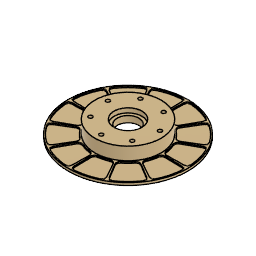
Brodie Stator Top (Autodesk Fusion 360 design; units mm, degrees)
Autodesk Fusion 360 part; units mm, degrees
sketch "Sketch1" plane through (0, 0, 0) normal (0, 0, 1) x (1, 0, 0)
  circle A0 centre (0, 0) radius 26
  circle A1 centre (0, 0) radius 47
  dimension "d1" = 52
  dimension "d2" = 94
  constraint coincident A0.centre A1.centre
  measures "d1" diameter of A0
  measures "d2" diameter of A1
extrude "Extrude1" add sketch "Sketch1" along normal blind 2 contours A0 | A1
sketch "Sketch2" plane through (0, 0, 2) normal (0, 0, 1) x (-1, 0, 0)
  circle A0 centre (0, 0) radius 47
  circle A1 centre (0, 0) radius 26
  constraint coincident A0.centre A1.centre
extrude "Extrude2" add sketch "Sketch2" along normal blind 10 contours A1
sketch "Sketch3" plane through (0, 0, 0) normal (0, 0, -1) x (1, 0, 0)
  circle A0 centre (0, 0) radius 47
  circle A1 centre (0, 0) radius 24
  constraint concentric A0 A1
extrude "Extrude3" cut sketch "Sketch3" against normal blind 3.5 contours A1
sketch "Sketch4" plane through (0, 0, 3.5) normal (0, 0, -1) x (1, 0, 0)
  circle A0 centre (0, 0) radius 24
  circle A1 centre (0, 0) radius 8.5
  dimension "d9" = 17
  constraint concentric A0 A1
  measures "d9" diameter of A1
extrude "Extrude4" cut sketch "Sketch4" against normal blind 31 contours A1
sketch "Sketch5" plane through (0, 0, 12) normal (0, 0, 1) x (-1, 0, 0)
  circle A0 centre (0, 0) radius 8.5
  circle A1 centre (0, 0) radius 26
  circle A2 centre (0, 0) radius 11
  constraint coincident A0.centre A1.centre
extrude "Extrude5" cut sketch "Sketch5" against normal blind 3.5 contours A2
sketch "Sketch6" plane through (0, 0, 3.5) normal (0, 0, -1) x (1, 0, 0)
  circle A0 centre (0, 0) radius 8.5
  circle A1 centre (0, 0) radius 24
  circle A2 centre (0, 0) radius 18
  constraint coincident A0.centre A1.centre
extrude "Extrude6" add sketch "Sketch6" along normal blind 1.5 contours A1
sketch "Sketch7" plane through (0, 0, 2) normal (0, 0, -1) x (1, 0, 0)
  circle A0 centre (0, 0) radius 18
  circle A1 centre (0, 0) radius 24
  circle A2 centre (0, 21) radius 1.5
  circle A3 centre (-16.4185, 13.0933) radius 1.5
  circle A4 centre (-20.4735, -4.6729) radius 1.5
  circle A5 centre (-9.1116, -18.9203) radius 1.5
  circle A6 centre (9.1116, -18.9203) radius 1.5
  circle A7 centre (20.4735, -4.6729) radius 1.5
  circle A8 centre (16.4185, 13.0933) radius 1.5
  dimension "d16" = 3
  dimension "d18" = 360
  measures "d16" diameter of A2
extrude "Extrude7" cut sketch "Sketch7" against normal blind 10 contours A2 | A3 | A4 | A5 | A6 | A7 | A8
sketch "Sketch8" plane through (0, 0, 2) normal (0, 0, 1) x (-1, 0, 0)
  circle A0 centre (0, 0) radius 26
  circle A1 centre (0, 0) radius 47
  line L0 (-0.5209, -29.8451) -> (-0.7486, -42.8887)
  line L1 (-14.4714, -26.1071) -> (-20.796, -37.517)
  arc A2 (-19.44, -41.6904) -> (-4.0097, -45.8249) centre (0, 0) ccw
  arc A3 (-10.6628, -24.8053) -> (-3.1684, -26.8134) centre (0, 0) ccw
  arc A4 (-4.0097, -45.8249) -> (-0.7486, -42.8887) centre (-3.7482, -42.8363) ccw
  arc A5 (-20.796, -37.517) -> (-19.44, -41.6904) centre (-18.1722, -38.9714) ccw
  arc A6 (-0.5209, -29.8451) -> (-3.1684, -26.8134) centre (-3.5205, -29.7927) ccw
  arc A7 (-10.6628, -24.8053) -> (-14.4714, -26.1071) centre (-11.8475, -27.5615) ccw
  arc A8 (-21.1397, -39.4118) -> (-20.8317, -40.3595) centre (-21.0253, -39.8985) ccw
  arc A9 (-2.139, -45.3682) -> (-1.3984, -44.7014) centre (-1.7408, -45.0658) ccw
  arc A10 (4.0097, -45.8249) -> (19.44, -41.6904) centre (0, 0) ccw
  arc A11 (0.7486, -42.8887) -> (4.0097, -45.8249) centre (3.7482, -42.8363) ccw
  arc A12 (1.3984, -44.7014) -> (2.139, -45.3682) centre (1.7408, -45.0658) ccw
  line L2 (0.5209, -29.8451) -> (0.7486, -42.8887)
  arc A13 (3.1684, -26.8134) -> (0.5209, -29.8451) centre (3.5205, -29.7927) ccw
  arc A14 (3.1684, -26.8134) -> (10.6628, -24.8053) centre (0, 0) ccw
  arc A15 (14.4714, -26.1071) -> (10.6628, -24.8053) centre (11.8475, -27.5615) ccw
  line L3 (14.4714, -26.1071) -> (20.796, -37.517)
  arc A16 (19.44, -41.6904) -> (20.796, -37.517) centre (18.1722, -38.9714) ccw
  arc A17 (20.8317, -40.3595) -> (21.1397, -39.4118) centre (21.0253, -39.8985) ccw
  arc A18 (26.3849, -37.6807) -> (37.6807, -26.3849) centre (0, 0) ccw
  arc A19 (22.0927, -36.7684) -> (26.3849, -37.6807) centre (24.6642, -35.2233) ccw
  arc A20 (23.5617, -38.0134) -> (24.5365, -38.2205) centre (24.0405, -38.1577) ccw
  line L4 (15.3737, -25.5861) -> (22.0927, -36.7684)
  arc A21 (16.1507, -21.6369) -> (15.3737, -25.5861) centre (17.9452, -24.041) ccw
  arc A22 (16.1507, -21.6369) -> (21.6369, -16.1507) centre (0, 0) ccw
  arc A23 (25.5861, -15.3737) -> (21.6369, -16.1507) centre (24.041, -17.9452) ccw
  line L5 (25.5861, -15.3737) -> (36.7684, -22.0927)
  arc A24 (37.6807, -26.3849) -> (36.7684, -22.0927) centre (35.2233, -24.6642) ccw
  arc A25 (38.2205, -24.5365) -> (38.0134, -23.5617) centre (38.1577, -24.0405) ccw
  arc A26 (41.6904, -19.44) -> (45.8249, -4.0097) centre (0, 0) ccw
  arc A27 (37.517, -20.796) -> (41.6904, -19.44) centre (38.9714, -18.1722) ccw
  arc A28 (39.4118, -21.1397) -> (40.3595, -20.8317) centre (39.8985, -21.0253) ccw
  line L6 (26.1071, -14.4714) -> (37.517, -20.796)
  arc A29 (24.8053, -10.6628) -> (26.1071, -14.4714) centre (27.5615, -11.8475) ccw
  arc A30 (24.8053, -10.6628) -> (26.8134, -3.1684) centre (0, 0) ccw
  arc A31 (29.8451, -0.5209) -> (26.8134, -3.1684) centre (29.7927, -3.5205) ccw
  line L7 (29.8451, -0.5209) -> (42.8887, -0.7486)
  arc A32 (45.8249, -4.0097) -> (42.8887, -0.7486) centre (42.8363, -3.7482) ccw
  arc A33 (45.3682, -2.139) -> (44.7014, -1.3984) centre (45.0658, -1.7408) ccw
  arc A34 (45.8249, 4.0097) -> (41.6904, 19.44) centre (0, 0) ccw
  arc A35 (42.8887, 0.7486) -> (45.8249, 4.0097) centre (42.8363, 3.7482) ccw
  arc A36 (44.7014, 1.3984) -> (45.3682, 2.139) centre (45.0658, 1.7408) ccw
  line L8 (29.8451, 0.5209) -> (42.8887, 0.7486)
  arc A37 (26.8134, 3.1684) -> (29.8451, 0.5209) centre (29.7927, 3.5205) ccw
  arc A38 (26.8134, 3.1684) -> (24.8053, 10.6628) centre (0, 0) ccw
  arc A39 (26.1071, 14.4714) -> (24.8053, 10.6628) centre (27.5615, 11.8475) ccw
  line L9 (26.1071, 14.4714) -> (37.517, 20.796)
  arc A40 (41.6904, 19.44) -> (37.517, 20.796) centre (38.9714, 18.1722) ccw
  arc A41 (40.3595, 20.8317) -> (39.4118, 21.1397) centre (39.8985, 21.0253) ccw
  arc A42 (37.6807, 26.3849) -> (26.3849, 37.6807) centre (0, 0) ccw
  arc A43 (36.7684, 22.0927) -> (37.6807, 26.3849) centre (35.2233, 24.6642) ccw
  arc A44 (38.0134, 23.5617) -> (38.2205, 24.5365) centre (38.1577, 24.0405) ccw
  line L10 (25.5861, 15.3737) -> (36.7684, 22.0927)
  arc A45 (21.6369, 16.1507) -> (25.5861, 15.3737) centre (24.041, 17.9452) ccw
  arc A46 (21.6369, 16.1507) -> (16.1507, 21.6369) centre (0, 0) ccw
  arc A47 (15.3737, 25.5861) -> (16.1507, 21.6369) centre (17.9452, 24.041) ccw
  line L11 (15.3737, 25.5861) -> (22.0927, 36.7684)
  arc A48 (26.3849, 37.6807) -> (22.0927, 36.7684) centre (24.6642, 35.2233) ccw
  arc A49 (24.5365, 38.2205) -> (23.5617, 38.0134) centre (24.0405, 38.1577) ccw
  arc A50 (19.44, 41.6904) -> (4.0097, 45.8249) centre (0, 0) ccw
  arc A51 (20.796, 37.517) -> (19.44, 41.6904) centre (18.1722, 38.9714) ccw
  arc A52 (21.1397, 39.4118) -> (20.8317, 40.3595) centre (21.0253, 39.8985) ccw
  line L12 (14.4714, 26.1071) -> (20.796, 37.517)
  arc A53 (10.6628, 24.8053) -> (14.4714, 26.1071) centre (11.8475, 27.5615) ccw
  arc A54 (10.6628, 24.8053) -> (3.1684, 26.8134) centre (0, 0) ccw
  arc A55 (0.5209, 29.8451) -> (3.1684, 26.8134) centre (3.5205, 29.7927) ccw
  line L13 (0.5209, 29.8451) -> (0.7486, 42.8887)
  arc A56 (4.0097, 45.8249) -> (0.7486, 42.8887) centre (3.7482, 42.8363) ccw
  arc A57 (2.139, 45.3682) -> (1.3984, 44.7014) centre (1.7408, 45.0658) ccw
  arc A58 (-4.0097, 45.8249) -> (-19.44, 41.6904) centre (0, 0) ccw
  arc A59 (-0.7486, 42.8887) -> (-4.0097, 45.8249) centre (-3.7482, 42.8363) ccw
  arc A60 (-1.3984, 44.7014) -> (-2.139, 45.3682) centre (-1.7408, 45.0658) ccw
  line L14 (-0.5209, 29.8451) -> (-0.7486, 42.8887)
  arc A61 (-3.1684, 26.8134) -> (-0.5209, 29.8451) centre (-3.5205, 29.7927) ccw
  arc A62 (-3.1684, 26.8134) -> (-10.6628, 24.8053) centre (0, 0) ccw
  arc A63 (-14.4714, 26.1071) -> (-10.6628, 24.8053) centre (-11.8475, 27.5615) ccw
  line L15 (-14.4714, 26.1071) -> (-20.796, 37.517)
  arc A64 (-19.44, 41.6904) -> (-20.796, 37.517) centre (-18.1722, 38.9714) ccw
  arc A65 (-20.8317, 40.3595) -> (-21.1397, 39.4118) centre (-21.0253, 39.8985) ccw
  arc A66 (-26.3849, 37.6807) -> (-37.6807, 26.3849) centre (0, 0) ccw
  arc A67 (-22.0927, 36.7684) -> (-26.3849, 37.6807) centre (-24.6642, 35.2233) ccw
  arc A68 (-23.5617, 38.0134) -> (-24.5365, 38.2205) centre (-24.0405, 38.1577) ccw
  line L16 (-15.3737, 25.5861) -> (-22.0927, 36.7684)
  arc A69 (-16.1507, 21.6369) -> (-15.3737, 25.5861) centre (-17.9452, 24.041) ccw
  arc A70 (-16.1507, 21.6369) -> (-21.6369, 16.1507) centre (0, 0) ccw
  arc A71 (-25.5861, 15.3737) -> (-21.6369, 16.1507) centre (-24.041, 17.9452) ccw
  line L17 (-25.5861, 15.3737) -> (-36.7684, 22.0927)
  arc A72 (-37.6807, 26.3849) -> (-36.7684, 22.0927) centre (-35.2233, 24.6642) ccw
  arc A73 (-38.2205, 24.5365) -> (-38.0134, 23.5617) centre (-38.1577, 24.0405) ccw
  arc A74 (-41.6904, 19.44) -> (-45.8249, 4.0097) centre (0, 0) ccw
  arc A75 (-37.517, 20.796) -> (-41.6904, 19.44) centre (-38.9714, 18.1722) ccw
  arc A76 (-39.4118, 21.1397) -> (-40.3595, 20.8317) centre (-39.8985, 21.0253) ccw
  line L18 (-26.1071, 14.4714) -> (-37.517, 20.796)
  arc A77 (-24.8053, 10.6628) -> (-26.1071, 14.4714) centre (-27.5615, 11.8475) ccw
  arc A78 (-24.8053, 10.6628) -> (-26.8134, 3.1684) centre (0, 0) ccw
  arc A79 (-29.8451, 0.5209) -> (-26.8134, 3.1684) centre (-29.7927, 3.5205) ccw
  line L19 (-29.8451, 0.5209) -> (-42.8887, 0.7486)
  arc A80 (-45.8249, 4.0097) -> (-42.8887, 0.7486) centre (-42.8363, 3.7482) ccw
  arc A81 (-45.3682, 2.139) -> (-44.7014, 1.3984) centre (-45.0658, 1.7408) ccw
  arc A82 (-45.8249, -4.0097) -> (-41.6904, -19.44) centre (0, 0) ccw
  arc A83 (-42.8887, -0.7486) -> (-45.8249, -4.0097) centre (-42.8363, -3.7482) ccw
  arc A84 (-44.7014, -1.3984) -> (-45.3682, -2.139) centre (-45.0658, -1.7408) ccw
  line L20 (-29.8451, -0.5209) -> (-42.8887, -0.7486)
  arc A85 (-26.8134, -3.1684) -> (-29.8451, -0.5209) centre (-29.7927, -3.5205) ccw
  arc A86 (-26.8134, -3.1684) -> (-24.8053, -10.6628) centre (0, 0) ccw
  arc A87 (-26.1071, -14.4714) -> (-24.8053, -10.6628) centre (-27.5615, -11.8475) ccw
  line L21 (-26.1071, -14.4714) -> (-37.517, -20.796)
  arc A88 (-41.6904, -19.44) -> (-37.517, -20.796) centre (-38.9714, -18.1722) ccw
  arc A89 (-40.3595, -20.8317) -> (-39.4118, -21.1397) centre (-39.8985, -21.0253) ccw
  arc A90 (-37.6807, -26.3849) -> (-26.3849, -37.6807) centre (0, 0) ccw
  arc A91 (-36.7684, -22.0927) -> (-37.6807, -26.3849) centre (-35.2233, -24.6642) ccw
  arc A92 (-38.0134, -23.5617) -> (-38.2205, -24.5365) centre (-38.1577, -24.0405) ccw
  line L22 (-25.5861, -15.3737) -> (-36.7684, -22.0927)
  arc A93 (-21.6369, -16.1507) -> (-25.5861, -15.3737) centre (-24.041, -17.9452) ccw
  arc A94 (-21.6369, -16.1507) -> (-16.1507, -21.6369) centre (0, 0) ccw
  arc A95 (-15.3737, -25.5861) -> (-16.1507, -21.6369) centre (-17.9452, -24.041) ccw
  line L23 (-15.3737, -25.5861) -> (-22.0927, -36.7684)
  arc A96 (-26.3849, -37.6807) -> (-22.0927, -36.7684) centre (-24.6642, -35.2233) ccw
  arc A97 (-24.5365, -38.2205) -> (-23.5617, -38.0134) centre (-24.0405, -38.1577) ccw
  dimension "d27" = 3
  dimension "d28" = 3
  dimension "d29" = 3
  dimension "d30" = 3
  dimension "d31" = 1
  dimension "d32" = 1
  dimension "d34" = 360
  constraint concentric A0 A3
  constraint tangent L0 A4
  constraint tangent A2 A4
  constraint tangent A2 A5
  constraint tangent L1 A5
  constraint tangent L0 A6
  constraint tangent A3 A6
  constraint tangent L1 A7
  constraint tangent A3 A7
  constraint midpoint A4 A9.centre
  constraint midpoint A5 A8.centre
  constraint coincident A5 A8.end
  constraint coincident A5 A8.start
  constraint coincident A4 A9.end
  constraint coincident A4 A9.start
  measures "d27" radius of A4
  measures "d28" radius of A5
  measures "d29" radius of A6
  measures "d30" radius of A7
  measures "d31" diameter of A9
  measures "d32" diameter of A8
extrude "Extrude8" cut sketch "Sketch8" against normal blind 1 contours L0 L1 A2 A3 A4 A5 A6 A7 | A4 A9 | A5 A8 | A10 A11 L2 A13 A14 A15 L3 A16 | A11 A12 | A16 A17 | A18 A19 L4 A21 A22 A23 L5 A24 | A19 A20 | A24 A25 | A74 A75 L18 A77 A78 A79 L19 A80 | A75 A76 | A80 A81 | A82 A83 L20 A85 A86 A87 L21 A88 | A83 A84 | A88 A89 | A90 A91 L22 A93 A94 A95 L23 A96 | A91 A92 | A96 A97
extrude "Extrude9" cut sketch "Sketch8" against normal blind 1 contours A26 A27 L6 A29 A30 A31 L7 A32 | A27 A28 | A32 A33 | A34 A35 L8 A37 A38 A39 L9 A40 | A35 A36 | A40 A41 | A42 A43 L10 A45 A46 A47 L11 A48 | A43 A44 | A48 A49 | A50 A51 L12 A53 A54 A55 L13 A56 | A51 A52 | A56 A57 | A58 A59 L14 A61 A62 A63 L15 A64 | A59 A60 | A64 A65 | A66 A67 L16 A69 A70 A71 L17 A72 | A67 A68 | A72 A73
